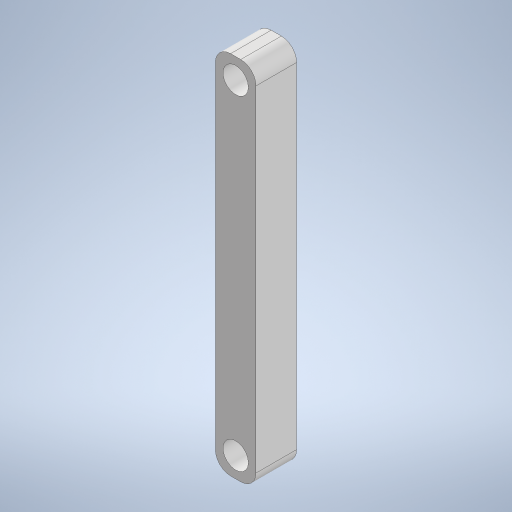
# Autodesk Inventor part: base
Saved by Autodesk Inventor 2024.1 (Build 281209000, 209)
## iProperties
Created: 2025-07-06
Part Number: base
Material: Generic
Document SubType Name: Modeling
Designer: iwheard
Density: 1 g/cm^3
Appearance: Default
Author: iwheard
Autodesk Inventor part; units mm, degrees
ref_plane "YZ Plane" through (0, 0, 0) normal (1, 0, 0) x (0, 1, 0)
ref_plane "XZ Plane" through (0, 0, 0) normal (0, 1, 0) x (-1, 0, 0)
ref_plane "XY Plane" through (0, 0, 0) normal (0, 0, 1) x (1, 0, 0)
sketch "Sketch1" plane through (0, 0, 0) normal (0, 0, 1) x (1, 0, 0)
  line L0 (0, 72) -> (8, 72)
  line L1 (8, 72) -> (8, 0)
  line L2 (8, 0) -> (0, 0)
  line L3 (0, 0) -> (0, 72)
  circle A0 centre (4, 68) radius 2.5
  circle A1 centre (4, 4) radius 2.5
  dimension "d0" = 8
  dimension "d1" = 72
  dimension "d2" = 5
  dimension "d3" = 5
  dimension "d4" = 4
  dimension "d5" = 64
  dimension "d7" = 4
  dimension "d8" = 4
  constraints: 8 end point, 2 centre point, 2 parallel, 1 coincident, 1 horizontal, 1 perpendicular, 1 vertical alignment
  measures "d0" distance between parallel lines of L3 L1
  measures "d1" distance between parallel lines of L2 L0
  measures "d2" diameter of A0
  measures "d3" diameter of A1
  measures "d4" distance from line of L0 A0.centre
  measures "d5" distance of A1.centre A0.centre
  measures "d7" distance from line of L2 A1.centre
  measures "d8" distance from line of L3 A0.centre
extrude "Extrusion1" add sketch "Sketch1" along normal blind 8
fillet "Fillet1" radius 3 4 edges at (8, 72, 4) (0, 72, 4) (8, 0, 4) (0, 0, 4)
equation "\"d3\" = d2"
body "Solid1"
